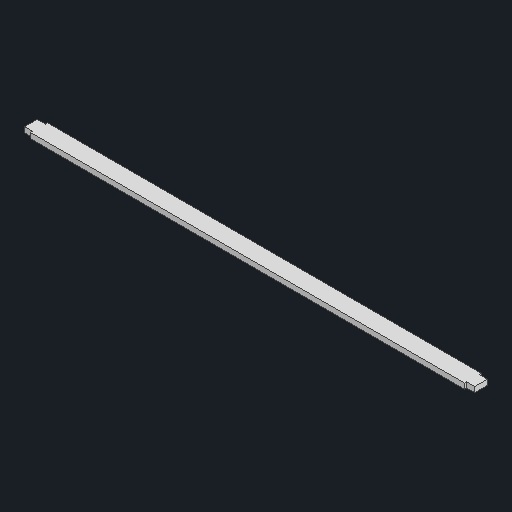
# Autodesk Inventor part: nose
Saved by Autodesk Inventor 2022.2 (Build 262287010, 287A)
## iProperties
Created: 2022-03-21
Part Number: nose
Material: Generic
Document SubType Name: Modeling
Designer: kardo
Density: 1 g/cm^3
Appearance: Default
Author: kardo
Autodesk Inventor part; units mm, degrees
ref_plane "YZ Plane" through (0, 0, 0) normal (1, 0, 0) x (0, 1, 0)
ref_plane "XZ Plane" through (0, 0, 0) normal (0, 1, 0) x (-1, 0, 0)
ref_plane "XY Plane" through (0, 0, 0) normal (0, 0, 1) x (1, 0, 0)
derived "parameters_frame.ipt"
derived "stencil_frame.ipt"
sketch "sk_joint_locations" plane through (81.12, 0, 0) normal (1, 0, 0) x (0, 1, 0)
  line L0 (0, 0) -> (135.09, 9.4464) construction
  line L1 (30.81, 28.832) -> (94.8, 28.832) construction
  arc A0 (30.81, 28.832) -> (9.48, 28.4869) centre (30.81, -630.4631) ccw construction
  line L2 (-254.1001, 19.9549) -> (9.48, 28.4869) construction
  line L3 (-363, 18.496) -> (-275.8801, 19.4795) construction
  arc A1 (-275.8801, 19.4795) -> (-254.1001, 19.9549) centre (-287.5515, 1053.3708) ccw construction
  line L4 (25.1322, 1581.9163) -> (267.6663, -1886.4825) construction
  line L5 (-242.0001, 1541.8302) -> (-242.0001, -1877.3857) construction
  line L6 (-120.9999, 1541.8302) -> (-120.9999, -1877.3857) construction
  line L7 (-363, 1541.8302) -> (-363, -1877.3857) construction
  line L8 (0, 1541.8302) -> (0, -1877.3857) construction
  line L9 (450.0665, 43.8884) -> (-613.9211, 6.7332) construction
  line L10 (-677.4829, -27.4989) -> (501.7293, 54.9597) construction
  line L11 (187.7215, 30.7247) -> (187.4423, 38.7198) construction
  line L12 (195.4031, 37.5588) -> (195.9625, 29.5588) construction
  line L13 (0, 3.808) -> (134.9306, 11.7256) construction
  line L14 (-242.0001, 45.8501) -> (-242.0001, 20.3465) construction
  line L15 (-363, 37.4293) -> (-363, 18.496) construction
  line L16 (-120.9999, 51.0063) -> (-120.9999, 24.2633) construction
  line L17 (0, 52.89) -> (0, 28.18) construction
  line L18 (132.2944, 49.425) -> (132.8217, 41.8851) construction
  line L19 (133.3489, 34.3453) -> (132.8217, 41.8851) construction
  line L20 (133.3489, 34.3453) -> (133.8761, 26.8054) construction
  line L21 (133.8761, 26.8054) -> (134.4034, 19.2655) construction
  line L22 (134.4034, 19.2655) -> (134.9306, 11.7256) construction
  line L23 (0, 3.808) -> (0, 0) construction
  line L24 (94.8, 37.536) -> (94.8, 28.832) construction
  line L25 (94.8, 35.548) -> (94.8, 30.82) construction
  spline S0 degree 4 poles (-363, 37.4293) (-272.3626, 45.1427) (-181.5879, 49.7528) (-90.8131, 52.89) (0, 52.89) knots 0 0 0 0 0 1 1 1 1 1
  spline S1 degree 3 poles (0, 52.89) (86.3106, 52.89) (181.3207, 49.5034) (237, 36.448) knots 0 0 0 0 1 1 1 1
  spline S2 degree 2 poles (135.09, 9.4464) (188.144, 13.1563) (237, 36.448) knots 0 0 0 1 1 1
  point P0 (187.5819, 34.7223)
  point P1 (195.6828, 33.5588)
  point P2 (134.9575, 11.3411)
  point P3 (-363, 27.9627)
  point P4 (-242.0001, 33.0983)
  point P5 (-120.9999, 37.6348)
  point P6 (0, 40.535)
  point P7 (94.8, 33.184)
derived "surface_body.ipt"
sketch "sk_long_inner" plane through (0, 0, 0) normal (1, 0, 0) x (0, 1, 0)
  line L0 (-483, 0) -> (357, 0) construction
  line L1 (-363, 107.6209) -> (-363, -224.5198) construction
  line L2 (-483, 54.4) -> (357, 54.4) construction
  line L3 (0, 107.6209) -> (0, -224.5198) construction
  line L4 (94.8, 107.6209) -> (94.8, -224.5198) construction
  line L5 (9.48, 28.832) -> (94.8, 28.832)
  line L6 (94.8, 37.536) -> (-363, 39.712)
  line L7 (9.48, 28.832) -> (-254.1001, 19.7253)
  line L8 (-254.1001, 19.7253) -> (-363, 18.496)
  line L9 (-363, 18.496) -> (94.8, 18.496) construction
  line L10 (94.8, 18.496) -> (94.8, 28.832) construction
  line L11 (-254.1001, 19.7253) -> (0, 18.496)
  line L12 (0, 18.496) -> (94.8, 28.832)
  line L13 (94.8, 37.536) -> (94.8, 28.832)
  line L14 (-120.9999, 107.6209) -> (-120.9999, -224.5198) construction
  line L15 (-242.0001, 107.6209) -> (-242.0001, -224.5198) construction
  point P0 (0, 0)
  point P1 (94.8, 23.664)
  point P2 (-363, 11.424)
ref_plane "plane_symmetry" through (0, 0, 0) normal (1, 0, 0) x (0, 1, 0)
ref_plane "plane_nose" through (0, 94.8, 0) normal (0, 1, 0) x (-1, 0, 0)
ref_plane "plane_tunnel_right" through (81.12, 0, 0) normal (1, 0, 0) x (0, 1, 0)
sketch "sk_nose_base" plane through (0, 94.8, 0) normal (0, 1, 0) x (-1, 0, 0)
  line L0 (0, -967.2299) -> (0, 1390.1376) construction
  line L1 (-81.12, -967.2299) -> (-81.12, 1390.1376) construction
  line L2 (-81.12, 36.336) -> (0, 36.336)
  line L3 (0, 36.336) -> (0, 30.032)
  line L4 (0, 30.032) -> (-81.12, 30.032)
  line L5 (-81.12, 30.032) -> (-81.12, 30.82)
  line L6 (-81.12, 30.82) -> (-84.12, 30.82)
  line L7 (-84.12, 30.82) -> (-84.12, 35.548)
  line L8 (-84.12, 35.548) -> (-81.12, 35.548)
  line L9 (-81.12, 35.548) -> (-81.12, 36.336)
  point P0 (0, 0)
  point P1 (0, 37.536)
  point P2 (0, 28.832)
  dimension "d3" = 3
  dimension "d6" = 1.2
  dimension "d7" = 1.2
  constraints: 16 end point, 6 collinear, 4 perpendicular, 2 point on line, 1 parallel
  measures "d3" distance between parallel lines of L7 L1
  measures "d6" distance from line of point (0, 37.536) L2
  measures "d7" distance from line of point (0, 28.832) L4
extrude "thicken" add sketch "sk_nose_base" against normal blind 2
mirror "mirror" about plane through (0, 0, 0) normal (1, 0, 0)
equation "\"d3\" = stringer_thickness"
equation "\"d6\" = shell_thickness"
equation "\"d7\" = shell_thickness"
equation "\"d4\" = bulkhead_thickness"
equation "\"stringer_thickness\" = 3"
equation "\"bulkhead_thickness\" = 2"
equation "\"shell_thickness\" = 1.2"
body "Solid1"
